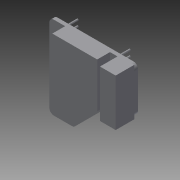
# Autodesk Inventor part: Adaptador TB6612FNG
Saved by Autodesk Inventor 2013 (Build 170138000, 138)
## iProperties
Created: 2013-05-03
Part Number: Adaptador TB6612FNG
Material: Generic
Document SubType Name: Modeling
Designer: otrab
Density: 1 g/cm^3
Author: otrab
Autodesk Inventor part; units mm, degrees
ref_plane "YZ Plane" through (0, 0, 0) normal (1, 0, 0) x (0, 1, 0)
ref_plane "XZ Plane" through (0, 0, 0) normal (0, 1, 0) x (-1, 0, 0)
ref_plane "XY Plane" through (0, 0, 0) normal (0, 0, 1) x (1, 0, 0)
sketch "Sketch1" plane through (0, 0, 0) normal (0, 1, 0) x (-1, 0, 0)
  line L0 (-2, 0) -> (-35.8284, 0)
  line L1 (-37.8284, -2) -> (-37.8284, -18)
  line L2 (-10, -37) -> (-2, -37)
  line L3 (0, -35) -> (0, -2)
  line L4 (-37, -36.9907) -> (-37, -19.9907) construction
  line L5 (-35.8284, -20) -> (-27.8284, -20)
  line L6 (0, -37) -> (-10, -37) construction
  line L7 (-11.4142, -36.4142) -> (-27.8284, -20)
  arc A0 (-37.8284, -18) -> (-35.8284, -20) centre (-35.8284, -18) ccw
  arc A1 (-35.8284, 0) -> (-37.8284, -2) centre (-35.8284, -2) ccw
  arc A2 (-2, -37) -> (0, -35) centre (-2, -35) ccw
  arc A3 (0, -2) -> (-2, 0) centre (-2, -2) ccw
  arc A4 (-11.4142, -36.4142) -> (-10, -37) centre (-10, -35) ccw
  point P0 (0, 0)
  point P1 (-37.8284, 0)
  point P2 (-37.8284, -20)
  dimension "d0" = 37
  dimension "d2" = 17
  dimension "d3" = 10
  dimension "d4" = 10
  dimension "d5" = 2
  dimension "d6" = 2
  constraints: 16 end point, 10 point on circle, 10 tangent, 8 point on line, 5 centre point, 3 equal radius, 3 parallel, 2 perpendicular, 1 horizontal
  measures "d0" distance of L6.start L4.start
  measures "d2" distance of L4.start L4.end
  measures "d3" distance of point (-37.828, -20) L5.end
  measures "d4" distance of L2.start L6.start
  measures "d5" radius of A0
  measures "d6" radius of A2
extrude "Extrusion1" add sketch "Sketch1" along normal blind 1.65
sketch "Sketch2" plane through (0, 0, 0) normal (0, -1, 0) x (1, 0, 0)
  line L0 (27.8284, -20) -> (35.8284, -20) projected
  line L1 (37.8284, -18) -> (37.8284, -2) projected
  line L2 (37.8105, 0.5) -> (30.8284, 0.5)
  line L3 (30.8284, 0.5) -> (30.8284, -20)
  line L4 (37.8105, -20.5) -> (37.8105, 0.5)
  line L5 (41.55, -10) -> (26.7279, -10) construction
  line L6 (37.8105, -20.5) -> (30.8284, -20.5)
  line L7 (30.8284, -20.5) -> (30.8284, -20)
  point P0 (0, 0)
  point P1 (37.8284, -10)
  dimension "d11" = 10.5
  constraints: 12 end point, 3 perpendicular, 2 parallel, 1 horizontal, 1 midpoint, 1 point on line, 1 other
  measures "d11" distance of L2.start point (37.828, -10)
extrude "Extrusion2" add sketch "Sketch2" along normal blind 8.3
sketch "Sketch3" plane through (0, 1.65, 0) normal (0, 1, 0) x (1, 0, 0)
  line L0 (0, 35) -> (0, 2) projected
  line L1 (2, 0) -> (35.8284, 0) projected
  line L2 (37.8284, 2) -> (37.8284, 18) projected
  line L3 (6, 38.3943) -> (6, -5.9246) construction
  line L4 (6, 0) -> (6, 1.25) construction
  circle A0 centre (6, 1.25) radius 0.37
  circle A1 centre (6, 3.85) radius 0.37
  circle A2 centre (6, 6.45) radius 0.37
  circle A3 centre (6, 9.05) radius 0.37
  circle A4 centre (6, 11.65) radius 0.37
  circle A5 centre (6, 14.25) radius 0.37
  circle A6 centre (6, 16.85) radius 0.37
  circle A7 centre (6, 19.45) radius 0.37
  circle A8 centre (6, 22.05) radius 0.37
  circle A9 centre (6, 24.65) radius 0.37
  circle A10 centre (6, 27.25) radius 0.37
  circle A11 centre (6, 29.85) radius 0.37
  circle A12 centre (6, 32.45) radius 0.37
  circle A13 centre (6, 35.05) radius 0.37
  line L5 (35.8284, 20) -> (27.8284, 20) projected
  line L6 (10, 37) -> (2, 37) projected
  line L7 (37.8284, 10) -> (29.2284, 10) construction
  line L8 (29.2284, 10) -> (29.2284, 28.7418) construction
  line L9 (29.2284, 20) -> (29.2284, 18.75) construction
  line L10 (29.2284, 0) -> (29.2284, 1.25) construction
  circle A14 centre (29.2284, 1.25) radius 0.37
  circle A15 centre (29.2284, 3.85) radius 0.37
  circle A16 centre (29.2284, 6.45) radius 0.37
  circle A17 centre (29.2284, 9.05) radius 0.37
  circle A18 centre (29.2284, 11.65) radius 0.37
  circle A19 centre (29.2284, 14.25) radius 0.37
  circle A20 centre (29.2284, 16.85) radius 0.37
  circle A21 centre (29.2284, 19.45) radius 0.37
  point P0 (0, 0)
  dimension "d16" = 1.25
  dimension "d17" = 0.74
  dimension "d20" = 2.6
  dimension "d27" = 8.6
  dimension "d37" = 0.74
  dimension "d40" = 2.6
  dimension "d50" = 6
  constraints: 22 centre point, 12 end point, 9 coincident, 7 point on line, 2 vertical, 1 collinear, 1 midpoint, 1 parallel, 1 perpendicular, 47 other
  measures "d16" distance of L4.start L4.end
  measures "d17" diameter of A0
  measures "d20" distance of A0.centre A1.centre
  measures "d27" distance of L7.start L7.end
  measures "d37" diameter of A14
  measures "d40" distance of L10.end point (29.228, 3.85)
  measures "d50" distance between parallel lines of L3 L0
extrude "Extrusion3" add sketch "Sketch3" along normal blind 5
sketch "Sketch4" plane through (0, 0, 0) normal (0, -1, 0) x (1, 0, 0)
  line L0 (30.8284, 0) -> (2, 0) projected
  line L1 (0, 0) -> (7, 0) construction
  line L2 (7, 0) -> (27, 0)
  line L3 (27, 0) -> (27, -20)
  line L4 (27, -20) -> (7, -20)
  line L5 (7, -20) -> (7, 0)
  dimension "d45" = 7
  dimension "d46" = 20
  dimension "d47" = 20
  constraints: 10 end point, 2 parallel, 1 horizontal, 1 perpendicular, 1 point on line
  measures "d45" distance of L1.start L1.end
  measures "d46" distance of L3.end L4.end
  measures "d47" distance of L4.end L1.end
extrude "Extrusion4" add sketch "Sketch4" along normal blind 5.7
equation "\"d47\" = d46"
body "Solid1"
